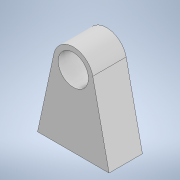
# Autodesk Inventor part: base
Saved by Autodesk Inventor 2021 (Build 250183000, 183)
## iProperties
Created: 2021-07-12
Part Number: base
Material: Genérico
Document SubType Name: Modeling
Designer: Leonardo Fabio Mercado Benítez
Density: 1 g/cm^3
Appearance: Valor por defecto
Author: Leonardo Fabio Mercado Benítez
Autodesk Inventor part; units mm, degrees
ref_plane "YZ Plane" through (0, 0, 0) normal (1, 0, 0) x (0, 1, 0)
ref_plane "XZ Plane" through (0, 0, 0) normal (0, 1, 0) x (-1, 0, 0)
ref_plane "XY Plane" through (0, 0, 0) normal (0, 0, 1) x (1, 0, 0)
sketch "Boceto1" plane through (0, 0, 0) normal (0, 0, 1) x (1, 0, 0)
  circle A0 centre (0, 0) radius 3.175
  arc A1 (4.0815, 0.8787) -> (-4.0815, 0.8787) centre (0, 0) ccw
  line L0 (0, 0) -> (0, -15) construction
  line L1 (0, -15) -> (7.5, -15) construction
  line L2 (0, -15) -> (-7.5, -15) construction
  line L3 (-7.5, -15) -> (-4.0815, 0.8787)
  line L4 (7.5, -15) -> (4.0815, 0.8787)
  line L5 (7.5, -15) -> (-7.5, -15)
  dimension "d0" = 6.35
  dimension "d1" = 1
  dimension "d2" = 15
  dimension "d3" = 7.5
  dimension "d4" = 7.5
  constraints: 12 end point, 2 centre point, 2 point on circle, 2 tangent, 1 coincident, 1 collinear, 1 horizontal, 1 perpendicular, 1 vertical
  measures "d0" diameter of A0
  measures "d1" radial gap between concentric circles of A0 A1
  measures "d2" distance of L0.start L0.end
  measures "d3" distance of L0.end L1.end
  measures "d4" distance of L0.end L2.end
extrude "Extrusión1" add sketch "Boceto1" along normal blind 7
